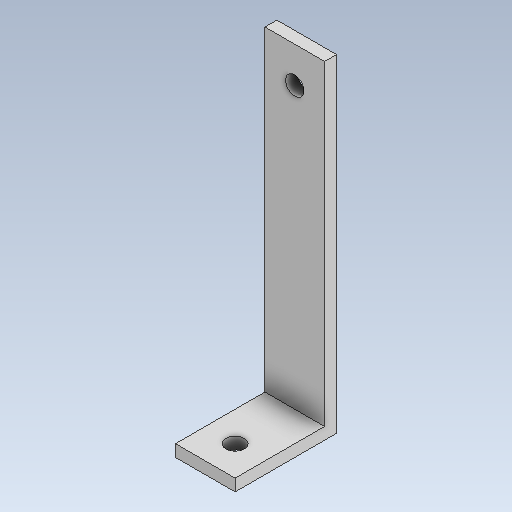
# Autodesk Inventor part: spacer tutup
Saved by Autodesk Inventor 2020 (Build 240168000, 168)
## iProperties
Created: 2020-03-26
Part Number: spacer tutup
Material: Generic
Document SubType Name: Modeling
Designer: ASUS
Density: 1 g/cm^3
Appearance: Default
Author: ASUS
Autodesk Inventor part; units mm, degrees
ref_plane "YZ Plane" through (0, 0, 0) normal (1, 0, 0) x (0, 1, 0)
ref_plane "XZ Plane" through (0, 0, 0) normal (0, 1, 0) x (-1, 0, 0)
ref_plane "XY Plane" through (0, 0, 0) normal (0, 0, 1) x (1, 0, 0)
sketch "Sketch1" plane through (0, 0, 0) normal (0, 0, 1) x (1, 0, 0)
  line L0 (5, -2) -> (-5, -2)
  line L1 (5, -2) -> (5, 53)
  line L2 (5, 53) -> (-5, 53)
  line L3 (-5, 53) -> (-5, -2)
  line L4 (0, 53) -> (0, 47)
  circle A0 centre (0, 47) radius 1.55
  point P0 (0, 0)
  dimension "d3" = 2
  dimension "d16" = 55
  dimension "d17" = 10
  dimension "d18" = 6
  dimension "d19" = 3.1
  constraints: 10 end point, 2 vertical, 1 centre point, 1 coincident, 1 horizontal, 1 midpoint, 1 perpendicular
  measures "d3" distance from line of point (0, 0) L0
  measures "d16" distance of L0.start L1.end
  measures "d17" distance of L1.end L2.end
  measures "d18" distance of L4.start L4.end
  measures "d19" diameter of A0
extrude "Extrusion1" add sketch "Sketch1" against normal blind 2
sketch "Sketch2" plane through (0, 0, 0) normal (0, 0, 1) x (1, 0, 0)
  line L0 (-5, 0) -> (5, 0)
  line L1 (5, 0) -> (5, -2)
  line L2 (5, -2) -> (-5, -2)
  line L3 (-5, -2) -> (-5, 0)
  point P0 (0, 0)
  constraints: 8 end point, 2 parallel, 1 horizontal, 1 perpendicular
extrude "Extrusion2" add sketch "Sketch2" along normal blind 15
sketch "Sketch3" plane through (-5, 0, 0) normal (0, 1, 0) x (1, 0, 0)
  circle A0 centre (5, -10) radius 1.55
  line L0 (10, -15) -> (0, -15) projected
  point P0 (5, 0)
  dimension "d11" = 3.1
  dimension "d15" = 5
  constraints: 1 centre point
  measures "d11" diameter of A0
  measures "d15" distance from line of L0 A0.centre
extrude "Extrusion3" cut sketch "Sketch3" against normal blind 2
body "Solid1"
